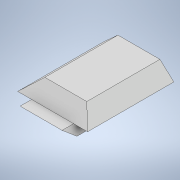
# Autodesk Inventor part: пример корпуса 1
Saved by Autodesk Inventor 2020.1 (Build 241239000, 239)
## iProperties
Created: 2021-12-15
Part Number: пример корпуса 1
Material: Типовые
Document SubType Name: Modeling
Designer: Ni3na
Density: 1 g/cm^3
Appearance: По умолчанию
Author: Ni3na
Autodesk Inventor part; units mm, degrees
ref_plane "YZ Plane" through (0, 0, 0) normal (1, 0, 0) x (0, 1, 0)
ref_plane "XZ Plane" through (0, 0, 0) normal (0, 1, 0) x (-1, 0, 0)
ref_plane "XY Plane" through (0, 0, 0) normal (0, 0, 1) x (1, 0, 0)
sketch "Эскиз2" plane through (0, 0, 0) normal (0, 0, 1) x (1, 0, 0)
  line L0 (104.717, 109.0836) -> (-45.283, 109.0836)
  line L1 (-45.283, 109.0836) -> (-45.283, 19.0836)
  line L2 (-45.283, 19.0836) -> (104.717, 19.0836)
  line L3 (104.717, 19.0836) -> (104.717, 109.0836)
  line L4 (-95.283, 19.0836) -> (154.717, 19.0836)
  line L5 (154.717, 19.0836) -> (154.717, 109.0836)
  line L6 (154.717, 109.0836) -> (-95.283, 109.0836)
  line L7 (-95.283, 109.0836) -> (-95.283, 19.0836)
  line L8 (154.717, 19.0836) -> (104.717, 19.0836)
  line L9 (104.717, 19.0836) -> (104.717, -10.9164)
  line L10 (104.717, -10.9164) -> (154.717, -10.9164)
  line L11 (154.717, -10.9164) -> (154.717, 19.0836)
  line L12 (-45.283, 19.0836) -> (-95.283, 19.0836)
  line L13 (-95.283, 19.0836) -> (-95.283, -10.9164)
  line L14 (-95.283, -10.9164) -> (-45.283, -10.9164)
  line L15 (-45.283, -10.9164) -> (-45.283, 19.0836)
  line L16 (-45.283, 64.0836) -> (-95.283, 64.0836)
  line L17 (-95.283, 64.0836) -> (-45.283, 109.0836)
  line L18 (104.717, 64.0836) -> (154.717, 64.0836)
  line L19 (154.717, 64.0836) -> (104.717, 109.0836)
  point P0 (0, 0)
  dimension "d0" = 150
  dimension "d1" = 50
  dimension "d2" = 50
  dimension "d3" = 30
  dimension "d4" = 90
  dimension "d5" = 0
  dimension "d6" = 0
  constraints: 40 end point, 8 parallel, 4 horizontal, 4 midpoint, 4 perpendicular
  measures "d0" distance of L1.end L2.end
  measures "d1" distance from line of L5 L0.start
  measures "d2" distance from line of L7 L0.end
  measures "d3" distance of L10.end L4.end
  measures "d4" distance of L4.start L6.end
  measures "d5" distance from line of L6 L0.end
  measures "d6" distance from line of L4 L1.end
extrude "Выдавливание1" add sketch "Эскиз2" along normal blind 350 contours L3 L2 L1 L0 | L19 L18 L3 | L1 L16 L17
sketch "Эскиз3" plane through (-45.283, 19.0836, 0) normal (-1, 0, 0) x (0, 0, 1)
  line L0 (0, 0) -> (350, 0) projected
  line L1 (296.6019, 0) -> (349.571, 44.6384)
  line L2 (350, 45) -> (350, 0) projected
  line L3 (349.571, 44.6384) -> (350, 45)
  line L4 (350, 45) -> (308.6701, 45)
  line L5 (0, 45) -> (350, 45) projected
  line L6 (308.6701, 45) -> (261.5284, 90)
  line L7 (0, 90) -> (350, 90) projected
  line L8 (0, 45) -> (0, 90) projected
  line L9 (350, 0) -> (0, 0)
  line L10 (0, 0) -> (0, 90)
  line L11 (0, 90) -> (350, 90)
  line L12 (350, 90) -> (350, 0)
  point P0 (0, -19.0836)
  constraints: 16 end point, 3 point on line, 2 parallel, 1 collinear, 1 horizontal, 1 perpendicular, 1 other
extrude "Выдавливание2" cut sketch "Эскиз3" against normal mid plane 1000 contours L1 L3 L2 L0 | L6 L7 L12 L4
